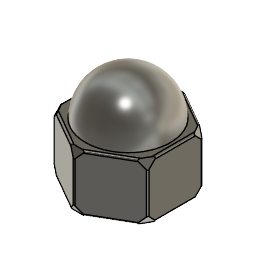
M3 Dome Nut (Autodesk Fusion 360 design; units mm, degrees)
Autodesk Fusion 360 part; units mm, degrees
sketch "Sketch1" plane through (0, 0, 0) normal (0, 0, 1) x (1, 0, 0)
  line L0 (-2.5, -1.4434) -> (0, -2.8868)
  line L1 (0, -2.8868) -> (2.5, -1.4434)
  line L2 (2.5, -1.4434) -> (2.5, 1.4434)
  line L3 (2.5, 1.4434) -> (0, 2.8868)
  line L4 (0, 2.8868) -> (-2.5, 1.4434)
  line L5 (-2.5, 1.4434) -> (-2.5, -1.4434)
  circle A0 centre (0, 0) radius 1.5
  dimension "d2" = 3
  constraint coincident A0.centre origin
  measures "d2" diameter of A0
extrude "Extrude1" add sketch "Sketch1" along normal blind 3
sphere "SpherePrimitive1" add diameter 4.5 placed x (-1, 0, 0) y (0, -1, 0) z (0, 0, 1) at (0, 0, 3)
extrude "Extrude2" cut sketch "Sketch1" along normal blind 4 contours A0
sketch "Sketch3" plane through (1.25, -2.1651, 0) normal (0.5, -0.866025, 0) x (0.866025, 0.5, 0)
  line L0 (-1.4434, 0) -> (1.4434, 0)
  line L1 (1.4434, 0) -> (1.4434, 3)
  line L2 (1.4434, 3) -> (-1.4434, 3)
  line L3 (-1.4434, 3) -> (-1.4434, 0)
  line L4 (-1.4434, 0) -> (-1.4434, 0.25)
  line L5 (-1.4434, 3) -> (-1.4434, 2.75)
  dimension "d10" = 0.25
  dimension "d11" = 0.25
  constraint coincident L0.start L3.end
  constraint perpendicular L0 L4
  constraint coincident L2.end L3.start
  constraint perpendicular L2 L5
  measures "d10" distance of L0.start L4.end
  measures "d11" distance of L2.end L5.end
sketch "Sketch4" plane through (0, 0, 3) normal (0, 0, 1) x (-1, 0, 0)
  circle A0 centre (0, 0) radius 2.25
  line L0 (2.5, -1.4434) -> (2.5, 1.4434)
  line L1 (2.5, 1.4434) -> (0, 2.8868)
  line L2 (0, 2.8868) -> (-2.5, 1.4434)
  line L3 (-2.5, 1.4434) -> (-2.5, -1.4434)
  line L4 (-2.5, -1.4434) -> (0, -2.8868)
  line L5 (0, -2.8868) -> (2.5, -1.4434)
  line L6 (0, 2.8868) -> (-0.2165, 2.7618)
  line L7 (0, 2.8868) -> (0.2165, 2.7618)
  dimension "d12" = 0.25
  dimension "d13" = 0.25
  constraint coincident L1.end L2.start
  constraint parallel L2 L6
  constraint parallel L1 L7
  measures "d12" distance of L1.end L6.end
  measures "d13" distance of L1.end L7.end
sketch "Sketch5" plane through (0, 0, 0) normal (0, 0, -1) x (1, 0, 0)
  line L0 (-2.5, 1.4434) -> (-2.5, -1.4434)
  line L1 (-2.5, -1.4434) -> (0, -2.8868)
  line L2 (0, -2.8868) -> (2.5, -1.4434)
  line L3 (2.5, -1.4434) -> (2.5, 1.4434)
  line L4 (2.5, 1.4434) -> (0, 2.8868)
  line L5 (0, 2.8868) -> (-2.5, 1.4434)
  line L6 (0, 2.8868) -> (0.2165, 2.7618)
  line L7 (0, 2.8868) -> (-0.2165, 2.7618)
  circle A0 centre (0, 0) radius 1.5
  dimension "d14" = 0.25
  dimension "d15" = 0.25
  constraint coincident L4.end L5.start
  constraint parallel L4 L6
  constraint parallel L5 L7
  measures "d14" distance of L4.end L6.end
  measures "d15" distance of L4.end L7.end
ref_plane "WorkPlane1" through (-0.2165, -2.7618, 0) normal (0, 0.894427, 0.447214) x (1, 0, 0)
ref_plane "WorkPlane2" through (-0.2165, -2.7618, 3) normal (0, 0.894427, -0.447214) x (-1, 0, 0)
sketch "Sketch6" plane through (0, -3.4094, 1.7047) normal (0, 0.894427, -0.447214) x (-1, 0, 0)
  line L0 (0.25, 1.5) -> (-0.25, 1.5)
  line L1 (-0.25, 1.5) -> (-0.25, 1.15)
  line L2 (-0.25, 1.15) -> (0.25, 1.15)
  line L3 (0.25, 1.15) -> (0.25, 1.5)
  constraint horizontal L0
  constraint vertical L1
  constraint horizontal L2
  constraint vertical L3
extrude "Extrude3" cut sketch "Sketch6" against normal blind 5
sketch "Sketch7" plane through (0, -2.2094, -1.1047) normal (0, 0.894427, 0.447214) x (1, 0, 0)
  line L0 (-0.3, -1.6) -> (0.3, -1.6)
  line L1 (0.3, -1.6) -> (0.3, -1.1)
  line L2 (0.3, -1.1) -> (-0.3, -1.1)
  line L3 (-0.3, -1.1) -> (-0.3, -1.6)
  constraint horizontal L0
  constraint vertical L1
  constraint horizontal L2
  constraint vertical L3
extrude "Extrude4" cut sketch "Sketch7" against normal blind 5
move_face "OffsetFaces1" offset -0.1 1 faces at (0, -2.8034, 2.9167)
move_face "OffsetFaces2" offset -0.1 1 faces at (0, -2.8034, 0.0833)
pattern_circular "C-Pattern1" count 6 over 360 about axis through (0, 0, 1.75) along (0, 0, 1) of 2 faces at (0, -2.7289, 0.1579) (0, -2.7289, 2.8421)
fillet "Fillet1" radius 0.1 18 edges at (0, -2.8868, 1.5) (-2.5, -1.4434, 1.5) (-2.5, 1.4434, 1.5) (0, 2.8868, 1.5) (2.5, 1.4434, 1.5) (2.5, -1.4434, 1.5) (2.5, 0, 3) (1.25, -2.1651, 3) (-1.25, -2.1651, 3) (-2.5, 0, 3) (-1.25, 2.1651, 3) (1.25, 2.1651, 3) (1.25, 2.1651, 0) (-1.25, 2.1651, 0) (-2.5, 0, 0) (-1.25, -2.1651, 0) (1.25, -2.1651, 0) (2.5, 0, 0)
thread "Thread2" "ISO Metric profile 3.0 M3x0.5 M3x0.5 6H" major diameter 3.086 minor diameter 2.529 pitch 0.5 angle 60 modelled right hand crest width 0.1368 on face at (1.4981, 0.0748, 1.3333) crest through (1.2645, 0, 0.125)
